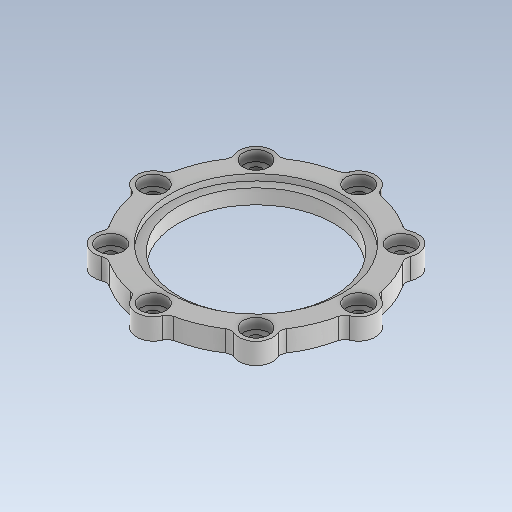
# Autodesk Inventor part: Outer_support_stand
Saved by Autodesk Inventor 2020 (Build 240168000, 168)
## iProperties
Created: 2021-09-25
Part Number: Outer_support_stand
Material: アルミニウム 2014-T4
Document SubType Name: Modeling
Designer: Masato Kubotera
Density: 2.8 g/cm^3
Appearance: 滑らか - 淡い灰色
Mass: 12.6488 g
Surface Area: 40.6204 cm^2
Volume: 4.51743 cm^3
Description: A2017 T5
Author: Masato Kubotera
Autodesk Inventor part; units mm, degrees
ref_plane "YZ Plane" through (0, 0, 0) normal (1, 0, 0) x (0, 1, 0)
ref_plane "XZ Plane" through (0, 0, 0) normal (0, 1, 0) x (-1, 0, 0)
ref_plane "XY Plane" through (0, 0, 0) normal (0, 0, 1) x (1, 0, 0)
derived "Trunk_horizontal_frame_01.ipt"
sketch "スケッチ1" plane through (0, 0, 0) normal (0, 0, 1) x (1, 0, 0)
  line L0 (-62, 30.75) -> (62, 30.75) projected
  line L1 (62, -30.75) -> (-62, -30.75) projected
  line L2 (-62, 30.75) -> (62, -30.75) construction
  line L3 (62, 30.75) -> (-62, -30.75) construction
  line L4 (0, 30.75) -> (0, -30.75) construction
  circle A0 centre (-44, 2.25) radius 10.5 construction
  line L5 (-57.5, 1.25) -> (-30.5, 1.25) construction
  line L6 (-30.5, 1.25) -> (-30.5, -25.75) construction
  line L7 (-30.5, -25.75) -> (-57.5, -25.75) construction
  line L8 (-57.5, -25.75) -> (-57.5, 1.25) construction
  line L9 (-44, 1.25) -> (-44, -25.75) construction
  line L10 (-57.5, -12.25) -> (-30.5, -12.25) construction
  circle A1 centre (-57.5, 1.25) radius 1.5 projected
  circle A2 centre (-57.5, -25.75) radius 1.5 projected
  circle A3 centre (-30.5, 1.25) radius 1.5 projected
  circle A4 centre (-30.5, -25.75) radius 1.5 projected
  line L11 (-27.5, 14.75) -> (-22.5, 14.75) construction
  line L12 (-22.5, 14.75) -> (-22.5, -10.25) construction
  line L13 (-22.5, -10.25) -> (-27.5, -10.25) construction
  line L14 (-27.5, -10.25) -> (-27.5, 14.75) construction
  line L15 (-27.5, 14.75) -> (-22.5, -10.25) construction
  line L16 (-22.5, 14.75) -> (-27.5, -10.25) construction
  line L17 (-27.55, 14.8) -> (-22.45, 14.8) projected
  line L18 (-22.45, 14.8) -> (-22.45, -10.3) projected
  line L19 (-22.45, -10.3) -> (-27.55, -10.3) projected
  line L20 (-27.55, -10.3) -> (-27.55, 14.8) projected
  line L21 (-27.55, 14.8) -> (-22.45, -10.3) construction
  line L22 (-22.45, 14.8) -> (-27.55, -10.3) construction
  line L23 (-27.55, 2.25) -> (-22.45, 2.25) construction
  line L24 (-25, 14.8) -> (-25, -10.3) construction
  arc A5 (-27.55, 14.8) -> (-27.55, 12.7) centre (-27.55, 13.75) ccw projected
  arc A6 (-22.45, 12.7) -> (-22.45, 14.8) centre (-22.45, 13.75) ccw projected
  arc A7 (-22.45, -10.3) -> (-22.45, -8.2) centre (-22.45, -9.25) ccw projected
  arc A8 (-27.55, -8.2) -> (-27.55, -10.3) centre (-27.55, -9.25) ccw projected
  circle A9 centre (-25, 27.75) radius 1.55 projected
  line L25 (-22.5, -17.25) -> (-27.5, -17.25) construction
  circle A10 centre (-25, -23.25) radius 1.55 projected
  circle A11 centre (-44, 2.25) radius 11 projected
  line L26 (62, 2.25) -> (-62, 2.25) construction
  line L27 (-60, 14.25) -> (-28, 14.25) construction
  line L28 (-28, 14.25) -> (-28, -28.75) construction
  line L29 (-28, -28.75) -> (-60, -28.75) construction
  line L30 (-60, -28.75) -> (-60, 14.25) construction
  line L31 (-60, 14.25) -> (-28, -28.75) construction
  line L32 (-28, 14.25) -> (-60, -28.75) construction
  line L33 (-62, 30.75) -> (-62, -30.75) construction
  line L34 (62, 30.75) -> (62, -30.75) construction
  circle A12 centre (-44, 2.25) radius 12.5 construction
  circle A13 centre (-44, 2.25) radius 20.5 construction
  circle A14 centre (-44, 2.25) radius 28.5 construction
  circle A15 centre (-44, 26.75) radius 1.25 construction
  circle A16 centre (-61.3241, 19.5741) radius 1.25 construction
  circle A17 centre (-68.5, 2.25) radius 1.25 construction
  circle A18 centre (-61.3241, -15.0741) radius 1.25 construction
  circle A19 centre (-44, -22.25) radius 1.25 construction
  circle A20 centre (-26.6759, -15.0741) radius 1.25 construction
  circle A21 centre (-19.5, 2.25) radius 1.25 construction
  circle A22 centre (-26.6759, 19.5741) radius 1.25 construction
  line L35 (-62, -21.122) -> (-62, -30.75) projected
  circle A23 centre (26.6759, -15.0741) radius 1.25 projected
  circle A24 centre (25, -23.25) radius 1.55 projected
  circle A25 centre (30.5, -25.75) radius 1.5 projected
  circle A26 centre (44, -22.25) radius 1.25 projected
  circle A27 centre (57.5, -25.75) radius 1.5 projected
  circle A28 centre (61.3241, -15.0741) radius 1.25 projected
  line L36 (62, -21.122) -> (62, -30.75) projected
  circle A29 centre (68.5, 2.25) radius 1.25 projected
  circle A30 centre (61.3241, 19.5741) radius 1.25 projected
  circle A31 centre (44, 26.75) radius 1.25 projected
  circle A32 centre (44, 2.25) radius 11 projected
  circle A33 centre (26.6759, 19.5741) radius 1.25 projected
  circle A34 centre (25, 27.75) radius 1.55 projected
  circle A35 centre (30.5, 1.25) radius 1.5 projected
  circle A36 centre (57.5, 1.25) radius 1.5 projected
  circle A37 centre (19.5, 2.25) radius 1.25 projected
  line L37 (22.45, -10.3) -> (27.55, -10.3) projected
  arc A38 (27.55, -10.3) -> (27.55, -8.2) centre (27.55, -9.25) ccw projected
  arc A39 (22.45, -8.2) -> (22.45, -10.3) centre (22.45, -9.25) ccw projected
  line L38 (22.45, 14.8) -> (22.45, -10.3) projected
  line L39 (27.55, -10.3) -> (27.55, 14.8) projected
  arc A40 (22.45, 14.8) -> (22.45, 12.7) centre (22.45, 13.75) ccw projected
  line L40 (27.55, 14.8) -> (22.45, 14.8) projected
  arc A41 (27.55, 12.7) -> (27.55, 14.8) centre (27.55, 13.75) ccw projected
  circle A42 centre (-44, 2.25) radius 20.51
  circle A43 centre (-44, 2.25) radius 18.5
  circle A44 centre (-44, 2.25) radius 28.5
  circle A45 centre (-44, 26.75) radius 1.55
  circle A46 centre (-61.3241, 19.5741) radius 1.55
  circle A47 centre (-68.5, 2.25) radius 1.55
  circle A48 centre (-61.3241, -15.0741) radius 1.55
  circle A49 centre (-44, -22.25) radius 1.55
  circle A50 centre (-26.6759, -15.0741) radius 1.55
  circle A51 centre (-19.5, 2.25) radius 1.55
  circle A52 centre (-26.6759, 19.5741) radius 1.55
  line L41 (-68.5, 2.25) -> (-73.5, 2.25) construction
  circle A53 centre (-26.6759, -15.0741) radius 6.25 construction
  circle A54 centre (-44, 2.25) radius 24.5 construction
  circle A55 centre (-44, 26.75) radius 3.05
  circle A56 centre (-61.3241, 19.5741) radius 3.05
  circle A57 centre (-68.5, 2.25) radius 3.05
  circle A58 centre (-44, -22.25) radius 3.05
  circle A59 centre (-26.6759, -15.0741) radius 3.05
  circle A60 centre (-19.5, 2.25) radius 3.05
  circle A61 centre (-26.6759, 19.5741) radius 3.05
  circle A62 centre (-61.3241, -15.0741) radius 3.05
  circle A63 centre (-30.5, -25.75) radius 2.4 projected
  arc A64 (-44, 30.75) -> (-47.969, 27.2469) centre (-44, 26.75) ccw
  arc A65 (-58.8689, 22.732) -> (-64.1525, 22.4025) centre (-61.3241, 19.5741) ccw
  arc A66 (-47.969, 27.2469) -> (-58.8689, 22.732) centre (-44, 2.25) ccw
  arc A67 (-64.1525, 22.4025) -> (-64.482, 17.1189) centre (-61.3241, 19.5741) ccw
  arc A68 (-64.482, 17.1189) -> (-68.9969, 6.219) centre (-44, 2.25) ccw
  arc A69 (-68.9969, 6.219) -> (-72.5, 2.25) centre (-68.5, 2.25) ccw
  arc A70 (-72.5, 2.25) -> (-68.9969, -1.719) centre (-68.5, 2.25) ccw
  arc A71 (-68.9969, -1.719) -> (-64.482, -12.6189) centre (-44, 2.25) ccw
  arc A72 (-64.482, -12.6189) -> (-64.1525, -17.9025) centre (-61.3241, -15.0741) ccw
  arc A73 (-64.1525, -17.9025) -> (-58.8689, -18.232) centre (-61.3241, -15.0741) ccw
  arc A74 (-58.8689, -18.232) -> (-47.969, -22.7469) centre (-44, 2.25) ccw
  arc A75 (-47.969, -22.7469) -> (-44, -26.25) centre (-44, -22.25) ccw
  arc A76 (-44, -26.25) -> (-40.031, -22.7469) centre (-44, -22.25) ccw
  arc A77 (-40.031, -22.7469) -> (-29.1311, -18.232) centre (-44, 2.25) ccw
  arc A78 (-29.1311, -18.232) -> (-23.8475, -17.9025) centre (-26.6759, -15.0741) ccw
  arc A79 (-23.8475, -17.9025) -> (-23.518, -12.6189) centre (-26.6759, -15.0741) ccw
  arc A80 (-23.518, -12.6189) -> (-19.0031, -1.719) centre (-44, 2.25) ccw
  arc A81 (-19.0031, -1.719) -> (-15.5, 2.25) centre (-19.5, 2.25) ccw
  arc A82 (-15.5, 2.25) -> (-19.0031, 6.219) centre (-19.5, 2.25) ccw
  arc A83 (-19.0031, 6.219) -> (-23.518, 17.1189) centre (-44, 2.25) ccw
  arc A84 (-23.518, 17.1189) -> (-23.8475, 22.4025) centre (-26.6759, 19.5741) ccw
  arc A85 (-23.8475, 22.4025) -> (-29.1311, 22.732) centre (-26.6759, 19.5741) ccw
  arc A86 (-29.1311, 22.732) -> (-40.031, 27.2469) centre (-44, 2.25) ccw
  arc A87 (-40.031, 27.2469) -> (-44, 30.75) centre (-44, 26.75) ccw
  arc A88 (-47.969, 27.2469) -> (-58.8689, 22.732) centre (-44, 2.25) ccw projected
  arc A89 (-44, 30.75) -> (-47.969, 27.2469) centre (-44, 26.75) ccw projected
  arc A90 (-58.8689, 22.732) -> (-64.482, 17.1189) centre (-61.3241, 19.5741) ccw projected
  arc A91 (-64.482, 17.1189) -> (-68.9969, 6.219) centre (-44, 2.25) ccw projected
  arc A92 (-68.9969, 6.219) -> (-68.9969, -1.719) centre (-68.5, 2.25) ccw projected
  arc A93 (-68.9969, -1.719) -> (-64.482, -12.6189) centre (-44, 2.25) ccw projected
  arc A94 (-64.482, -12.6189) -> (-62, -19.0166) centre (-61.3241, -15.0741) ccw projected
  line L42 (-62, -19.0166) -> (-62, -21.122) projected
  arc A95 (47.969, 27.2469) -> (44, 30.75) centre (44, 26.75) ccw projected
  arc A96 (58.8689, 22.732) -> (47.969, 27.2469) centre (44, 2.25) ccw projected
  arc A97 (64.482, 17.1189) -> (58.8689, 22.732) centre (61.3241, 19.5741) ccw projected
  arc A98 (68.9969, 6.219) -> (64.482, 17.1189) centre (44, 2.25) ccw projected
  arc A99 (68.9969, -1.719) -> (68.9969, 6.219) centre (68.5, 2.25) ccw projected
  arc A100 (64.482, -12.6189) -> (68.9969, -1.719) centre (44, 2.25) ccw projected
  arc A101 (62, -19.0166) -> (64.482, -12.6189) centre (61.3241, -15.0741) ccw projected
  line L43 (62, -19.0166) -> (62, -21.122) projected
  line L44 (19.5, 25.75) -> (-19.5, 25.75) projected
  line L45 (-19.5, 25.75) -> (-19.5, 7.25) projected
  circle A102 centre (-25, 27.75) radius 2.75 construction
  line L46 (-15.1699, 4.75) -> (15.1699, 4.75) projected
  arc A103 (-15.1699, 4.75) -> (-19.5, 7.25) centre (-19.5, 2.25) ccw projected
  line L47 (19.5, 25.75) -> (19.5, 7.25) projected
  arc A104 (19.5, 7.25) -> (15.1699, 4.75) centre (19.5, 2.25) ccw projected
  arc A105 (-19.5, -2.75) -> (-15.1699, -0.25) centre (-19.5, 2.25) ccw projected
  line L48 (-15.1699, -0.25) -> (15.1699, -0.25) projected
  arc A106 (15.1699, -0.25) -> (19.5, -2.75) centre (19.5, 2.25) ccw projected
  line L49 (-19.5, -2.75) -> (-19.5, -25.75) projected
  line L50 (-19.5, -25.75) -> (19.5, -25.75) projected
  line L51 (19.5, -25.75) -> (19.5, -2.75) projected
  point P0 (0, 0)
  point P1 (-25, 2.25)
  point P2 (-44, -7.25)
  point P3 (-23.326, 21.76)
  point P4 (-23.2248, 21.76)
  point P5 (-23.8475, 22.4025)
  point P6 (-64.1525, -17.9025)
  point P7 (-44, -26.25)
  point P8 (-23.8475, -17.9025)
  point P9 (-15.5, 2.25)
  point P10 (-23.8475, 22.4025)
  point P11 (-25, 2.25)
  point P12 (27.9147, 19.7411)
  point P13 (27.51, 18.6431)
  point P14 (27.55, -8.2)
  point P15 (-27.51, 18.6431)
  point P16 (-27.9147, 19.7411)
  point P17 (-26.4271, 21.76)
  point P18 (-26.9247, 21.76)
  point P19 (-27.51, 20.5051)
  point P20 (27.51, 20.5051)
  point P21 (26.9247, 21.76)
  point P22 (26.4271, 21.76)
  point P23 (-47, 30.75)
  point P24 (47, 30.75)
  dimension "d2" = 0.01
  dimension "d3" = 37
  dimension "d4" = 3.1
  dimension "d5" = 3.1
  dimension "d6" = 3.1
  dimension "d7" = 3.1
  dimension "d8" = 3.1
  dimension "d9" = 3.1
  dimension "d10" = 3.1
  dimension "d11" = 3.1
  dimension "d16" = 6.1
  dimension "d17" = 6.1
  dimension "d18" = 6.1
  dimension "d20" = 6.1
  dimension "d21" = 6.1
  dimension "d22" = 6.1
  dimension "d23" = 6.1
  dimension "d24" = 6.1
  dimension "d27" = 4.8
  dimension "d30" = 360
  constraints: 48 point on circle, 42 centre point, 19 coincident, 1 vertical alignment, 88 other
  measures "d2" radial gap between concentric circles of A13 A42
  measures "d3" diameter of A43
  measures "d4" diameter of A45
  measures "d5" diameter of A46
  measures "d6" diameter of A47
  measures "d7" diameter of A48
  measures "d8" diameter of A49
  measures "d9" diameter of A50
  measures "d10" diameter of A51
  measures "d11" diameter of A52
  measures "d16" diameter of A55
  measures "d17" diameter of A56
  measures "d18" diameter of A57
  measures "d20" diameter of A58
  measures "d21" diameter of A59
  measures "d22" diameter of A60
  measures "d23" diameter of A61
  measures "d24" diameter of A62
  measures "d27" radial gap between concentric circles of A42 A66
extrude "押し出し1" add sketch "スケッチ1" along normal blind 5 contours A87 A86 A85 A84 A83 A6 L17 A5 A42 A8 L19 A7 A80 A79 A78 A77 A76 A75 A74 A73 A72 A71 A70 A69 A68 A67 A65 A66 A64 | L45 A103 A83 A82 A81 A80 A105 L49 A7 L18 A60 A6 | A83 A103 L45 | A83 A6 L18 | L18 A60 L19 L20 A42 L17 | L20 A42 A5 | A80 L49 A105 | A42 L20 A8 | A80 A7 L18 picked at (-27.6201, 14.693) picked at (-27.6201, -10.193)
extrude "押し出し2" add sketch "スケッチ1" along normal blind 3.5 contours A42 L20 A43 | L20 A5 A42 | A5 L20 A43 A8 A42 | A8 L20 A42 picked at (-27.6349, 13.3104) picked at (-27.6349, -8.8104)
extrude "押し出し3" add sketch "スケッチ1" along normal blind 2.5 contours A60 L18 | L18 A60 | A55 | A56 | A57 | A58 | A59 | A61 | A62
fillet "フィレット1" radius 2 16 edges at (-40.031, -22.7469, 2.5) (-29.1311, -18.232, 2.5) (-23.518, -12.6189, 2.5) (-19.0031, -1.719, 2.5) (-19.0031, 6.219, 2.5) (-23.518, 17.1189, 2.5) (-29.1311, 22.732, 2.5) (-40.031, 27.2469, 2.5) (-58.8689, 22.732, 2.5) (-68.9969, 6.219, 2.5) (-47.969, 27.2469, 2.5) (-64.482, 17.1189, 2.5) (-68.9969, -1.719, 2.5) (-64.482, -12.6189, 2.5) (-47.969, -22.7469, 2.5) (-58.8689, -18.232, 2.5)
equation "\"d5\" = d4"
equation "\"d6\" = d4"
equation "\"d7\" = d4"
equation "\"d8\" = d4"
equation "\"d9\" = d4"
equation "\"d10\" = d4"
equation "\"d11\" = d4"
equation "\"d17\" = d16"
equation "\"d18\" = d16"
equation "\"d20\" = d16"
equation "\"d21\" = d16"
equation "\"d22\" = d16"
equation "\"d23\" = d16"
equation "\"d24\" = d16"
